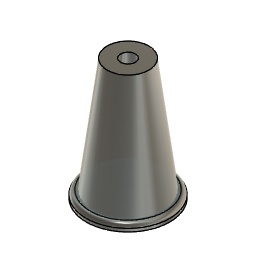
cono maniglia garage (Autodesk Fusion 360 design; units mm, degrees)
Autodesk Fusion 360 part; units mm, degrees
note: some values were not read from the file. Chosen so that the rebuilt part matches the saved one: which sketch regions a step uses; add or cut.
sketch "Schizzo2" plane through (0, 0, 0) normal (0, 0, 1) x (1, 0, 0)
  circle A0 centre (0, 0) radius 20
  circle A1 centre (0, 0) radius 10
  circle A2 centre (0, 0) radius 17.5
  dimension "d6" = 40
  dimension "d7" = 20
  dimension "d8" = 35
  constraint coincident A0.centre A1.centre
  constraint concentric A0 A1
  constraint concentric A1 A2
  measures "d6" diameter of A0
  measures "d7" diameter of A1
  measures "d8" diameter of A2
sketch "Schizzo3" plane through (0, 0, 0) normal (0, 0, 1) x (1, 0, 0)
  circle A0 centre (0, 0) radius 20
  circle A1 centre (0, 0) radius 17.5
  circle A2 centre (0, 0) radius 10
  dimension "d11" = 40
  dimension "d12" = 35
  dimension "d13" = 20
  constraint coincident A0.centre A1.centre
  constraint concentric A0 A1
  constraint concentric A1 A2
  measures "d11" diameter of A0
  measures "d12" diameter of A1
  measures "d13" diameter of A2
sketch "Schizzo4" plane through (0, 0, 58) normal (0, 0, 1) x (-1, 0, 0)
  circle A0 centre (0, 0) radius 10
  circle A1 centre (0, 0) radius 17.5
  circle A2 centre (0, 0) radius 3.5
  circle A3 centre (0, 0) radius 10
  dimension "d16" = 7
  dimension "d17" = 20
  constraint concentric A0 A2
  constraint concentric A2 A3
  measures "d16" diameter of A2
  measures "d17" diameter of A3
loft "Loft1" add profiles "Schizzo2", "Schizzo4" section 1 contours A1 | A2 section 2 contours A0 A3 makes body 1
extrude "Estrusione4" cut sketch "Schizzo2" along normal blind 7 contours A1 bodies 1
extrude "Estrusione5" cut 1 faces at (14.9348, -0.8694, 0) along direction (0, 0, -1) blind 1 on bodies 1 bodies 1
extrude "Estrusione6" add 1 faces at (3.1852, -0.9825, 7) along direction (0, 0, -1) blind 7 on bodies 1 bodies 1
loft "Loft2" cut profiles "Schizzo4", "Schizzo2" section 1 contours A2 section 2 contours A1 bodies 1
extrude "Estrusione7" add sketch "Schizzo2" along normal blind 3.5 separate body contours A0 makes body 2
move_face "FacceDiOffset1" offset 1 1 faces at (17.4782, -0.8723, 1.1667) on bodies 2
fillet "Raccordo1" radius 2 1 edges at (-18.6465, -7.2323, 3.5) on bodies 2
copy_body "Corpo->Comp1" bodies 2 removing the originals makes body 3 in component "Component"
copy_body "Corpo->Comp2" bodies 1 removing the originals makes body 4 in component "Component'"
sketch "Schizzo5" plane through (0, 0, 3.5) normal (0, 0, 1) x (-1, 0, 0)
  circle A0 centre (0, 0) radius 16.5
  circle A1 centre (0, 0) radius 18
fillet "Raccordo1'" [suppressed] in component "Component'"
fillet "Raccordo1''" [suppressed] in component "Component"
component "Component" placed x (1, 0, 0) y (0, 1, 0) z (0, 0, 1) at (0, 0, 0)
component "Component'" placed x (1, 0, 0) y (0, 1, 0) z (0, 0, 1) at (0, 0, 0)
